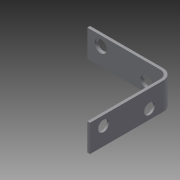
# Autodesk Inventor part: 30mmCornerBracket
Saved by Autodesk Inventor 2015 (Build 190159000, 159)
## iProperties
Created: 2015-04-22
Part Number: 30mmCornerBracket
Material: Generic
Document SubType Name: Modeling
Designer: krosie
Density: 1 g/cm^3
Appearance: Default
Author: krosie
Autodesk Inventor part; units mm, degrees
ref_plane "YZ Plane" through (0, 0, 0) normal (1, 0, 0) x (0, 1, 0)
ref_plane "XZ Plane" through (0, 0, 0) normal (0, 1, 0) x (-1, 0, 0)
ref_plane "XY Plane" through (0, 0, 0) normal (0, 0, 1) x (1, 0, 0)
sketch "Sketch1" plane through (0, 0, 0) normal (0, 0, 1) x (1, 0, 0)
  line L0 (0, 0) -> (27, 0)
  line L1 (30, -3) -> (30, -30)
  arc A0 (30, -3) -> (27, 0) centre (27, -3) ccw
  point P0 (30, 0)
  dimension "d0" = 30
  dimension "d1" = 30
  dimension "d7" = 3
  constraints: 4 end point, 2 point on circle, 2 point on line, 2 tangent, 1 centre point, 1 horizontal, 1 perpendicular
  measures "d0" distance of L0.start point (30, 0)
  measures "d1" distance of point (30, 0) L1.end
  measures "d7" radius of A0
sketch "Sketch2" plane through (0, 0, 0) normal (1, 0, 0) x (0, 1, 0)
  line L0 (0, 0) -> (0, -10)
  line L1 (0, -10) -> (1, -10)
  line L2 (1, -10) -> (1, 0)
  line L3 (1, 0) -> (0, 0)
  dimension "d2" = 10
  dimension "d3" = 1
  dimension "d4" = 10
  constraints: 8 end point, 2 perpendicular, 1 vertical
  measures "d2" distance of L0.start L0.end
  measures "d3" distance of L0.end L1.end
  measures "d4" distance of L1.end L2.end
sweep "Sweep1" add profiles "Sketch2" path "Sketch1"
hole "Hole1" at (5, 1, -3.5) direction (0, -1, 0) diameter 4 end through all
hole "Hole2" at (22, 1, -6.5) direction (0, -1, 0) diameter 4 end through all
hole "Hole3" at (31, -8, -6.5) direction (-1, 0, 0) diameter 4 end through all
hole "Hole4" at (31, -25, -3.5) direction (-1, 0, 0) diameter 4 end through all
chamfer "Chamfer1" distance 0.25 angle 45 4 edges at (5, 0, -5.5) (22, 0, -8.5) (30, -8, -4.5) (30, -25, -1.5)
body "Solid1"
